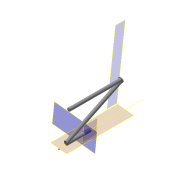
# Autodesk Inventor part: cellSTORM_lightpath
Saved by Autodesk Inventor 2022 (Build 260153000, 153)
## iProperties
Created: 2020-04-25
Part Number: cellSTORM_lightpath
Material: Generic
Document SubType Name: Modeling
Designer: diederichbenedict
Density: 1 g/cm^3
Appearance: Default
Author: diederichbenedict
Autodesk Inventor part; units mm, degrees
ref_plane "YZ Plane" through (0, 0, 0) normal (1, 0, 0) x (0, 1, 0)
ref_plane "XZ Plane" through (0, 0, 0) normal (0, 1, 0) x (-1, 0, 0)
ref_plane "XY Plane" through (0, 0, 0) normal (0, 0, 1) x (1, 0, 0)
ref_plane "Work Plane1" through (-18.0552, 1.9841, 10) normal (0, 0, -1) x (-0.994, 0.1092, 0)
ref_plane "Work Plane4" through (0, 0, 10) normal (-0.994, 0.1092, 0) x (-0.1092, -0.994, 0)
ref_plane "Work Plane3" through (-40.2485, 19.0101, 10) normal (-0.994, 0.1092, 0) x (-0.1092, -0.994, 0)
sketch "Sketch1" plane through (0, 0, 10) normal (-0.994, 0.1092, 0) x (-0.1092, -0.994, 0)
  line L0 (0, -10) -> (0, 30)
  line L1 (0, 30) -> (-50, -56.6025)
  line L2 (-50, -56.6025) -> (-50, 28.3975)
  line L3 (-7.1094, 32.5876) -> (7.1094, 27.4124)
  line L4 (-58.0583, -53.6696) -> (-41.9417, -59.5355)
  line L5 (-50, -56.6025) -> (-68.7133, -89.015)
  line L6 (-65.9988, -87.2149) -> (-113.9988, -87.2149)
  line L7 (-85.9997, -87.615) -> (-57.6047, -87.615)
  line L8 (-57.6047, -90.815) -> (-85.9997, -90.815)
  line L9 (-81.8462, -89.015) -> (-68.7133, -89.015)
  dimension "d0" = 40
  dimension "d1" = 100
  dimension "d2" = 30
  dimension "d3" = 85
  dimension "d4" = 30
  dimension "d6" = 70
  dimension "d19" = 1.4
  constraints: 21 end point, 2 midpoint, 2 parallel, 1 collinear, 1 horizontal, 1 vertical, 9 other
  measures "d0" distance of L0.end L0.start
  measures "d1" distance of L0.end L1.end
  measures "d2" angle of L1 L0
  measures "d3" distance of L1.end L2.end
  measures "d4" angle of L1 L2
  measures "d6" angle of L3 L0
  measures "d19" vertical distance of L5.end L7.end
ref_plane "Work Plane7" through (-18.0552, 1.9841, 10) normal (0, 0, -1) x (-0.994, 0.1092, 0)
sketch "Sketch3" plane through (-18.0552, 1.9841, 10) normal (0, 0, -1) x (-0.994, 0.1092, 0)
  circle A0 centre (-18.1638, 0) radius 11.5 projected
  circle A1 centre (-18.1638, 0) radius 2.5
  point P0 (-18.1638, 0)
  dimension "d7" = 5
  constraints: 1 centre point, 1 coincident
  measures "d7" diameter of A1
sweep "Sweep1" add profiles "Sketch3" path "Sketch1" path curves L0 L1 L2 contours A1
ref_plane "Work Plane8" through (-22.055, 95.458, -62.5) normal (-0.994, 0.1092, 0) x (-0.1092, -0.994, 0)
sketch "Sketch4" plane through (-22.055, 95.458, -62.5) normal (-0.994, 0.1092, 0) x (-0.1092, -0.994, 0)
  line L0 (44.9778, 100.8975) -> (39.9778, 100.8975) projected
  line L1 (42.4778, 15.8975) -> (42.4778, 15.8975) projected
  line L2 (42.4778, 15.8975) -> (42.4778, 15.8975) projected
  line L3 (42.4778, 15.8975) -> (42.4778, 15.8975) projected
  line L4 (42.4778, 15.8975) -> (42.4778, 15.8975) projected
  line L5 (92.4778, 102.5) -> (92.4778, 102.5) projected
  line L6 (92.4778, 102.5) -> (92.4778, 102.5) projected
  line L7 (92.4778, 102.5) -> (92.4778, 102.5) projected
  line L8 (92.4778, 102.5) -> (92.4778, 102.5) projected
  line L9 (94.9778, 62.5) -> (89.9778, 62.5) projected
  line L10 (56.4279, -3) -> (16.4279, -3) projected
  line L11 (39.9778, 6.5673) -> (39.9778, 100.8975) projected
  line L12 (44.9778, 25.2276) -> (44.9778, 100.8975) projected
  line L13 (94.9778, 111.8301) -> (44.9778, 25.2276) projected
  line L14 (89.9778, 93.1699) -> (39.9778, 6.5673) projected
  line L15 (89.9778, 62.5) -> (89.9778, 93.1699) projected
  line L16 (94.9778, 62.5) -> (94.9778, 111.8301) projected
  line L17 (34.8879, 19.8987) -> (57.029, 15.9946)
  line L18 (57.029, 15.9946) -> (43.097, -3.4007)
  line L19 (43.097, -3.4007) -> (27.2737, 11.5768)
  line L20 (27.2737, 11.5768) -> (33.0712, 21.6183)
  line L21 (34.8879, 19.8987) -> (33.0712, 21.6183)
  line L22 (80.9168, 101.8756) -> (102.3497, 98.0964)
  line L23 (102.3497, 98.0964) -> (104.1096, 108.0773)
  line L24 (104.1096, 108.0773) -> (90.6818, 110.445)
  line L25 (90.6818, 110.445) -> (80.9168, 101.8756)
  point P0 (92.4778, 62.5)
  dimension "d10" = 70
  dimension "d11" = 7
  dimension "d12" = 7
  constraints: 18 end point, 2 parallel, 1 perpendicular, 1 point on line
  measures "d10" angle of L17 L14
  measures "d11" distance from line of L17 L12.start
  measures "d12" distance from line of L22 L15.end
extrude "Extrusion1" cut sketch "Sketch4" against normal through all contours L17 L14 L11 | L11 L14 L17 L18 L10 L19 L20 L21 | L22 L25 L24 L13 | L13 L24 L16 L22 | L16 L24 L23 L22 | L18 L19 L10
sketch "Sketch5" plane through (5.4615, 49.7008, -43.9396) normal (0.019, 0.1726, -0.9848) x (-0.994, 0.1092, 0)
  ellipse E0 centre (0, -1.4169) end of major axis (0, -4.0774) minor radius 2.5 (-2.4054, -0.6919) -> (2.4054, -0.6919) ccw projected
  ellipse E1 centre (0, 0) end of major axis (0, 2.5386) minor radius 2.5 (2.4054, -0.6919) -> (-2.4054, -0.6919) ccw projected
  line L0 (-2.4054, -0.1127) -> (2.4054, -0.1127) projected
  circle A0 centre (0, -0.1127) radius 3.7871
  point P0 (0, -41.6104)
  constraints: 1 centre point, 4 other
extrude "Extrusion2" add sketch "Sketch5" against normal blind 1 contours E1 E0 A0 | E0 A0 E1
sketch "Sketch6" plane through (0.1524, 1.3871, 37.5831) normal (-0.019, -0.1726, 0.9848) x (0.994, -0.1092, 0)
  ellipse E0 centre (0, 0) end of major axis (0, -2.6604) minor radius 2.5 (2.4054, -0.7251) -> (-2.4054, -0.7251) ccw projected
  ellipse E1 centre (0, -1.4169) end of major axis (0, 1.1216) minor radius 2.5 (-2.4054, -0.7251) -> (2.4054, -0.7251) ccw projected
  line L0 (-2.4054, -0.1127) -> (2.4054, -0.1127) projected
  circle A0 centre (0, -0.1127) radius 3.2394
  point P0 (0, -7.9004)
  constraints: 1 centre point, 4 other
extrude "Extrusion3" add sketch "Sketch6" against normal blind 1 contours E1 A0 E0 | E0 E1 A0
ref_plane "Arbeitsebene10" through (0, 0, 0) normal (0.1092, 0.994, 0) x (0, 0, -1)
ref_plane "Arbeitsebene9" through (28.1562, 85.4859, 52.7288) normal (0.1092, 0.994, 0) x (0, 0, -1)
sketch "Skizze7" plane through (0, 0, 0) normal (1, 0, 0) x (0, 1, 0)
  ellipse E0 centre (1.916, 36.6615) end of major axis (-0.7027, 36.2019) minor radius 0.0475 (1.1885, 36.4876) -> (0.6825, 36.4876) ccw projected
  ellipse E1 centre (0, 40) end of major axis (2.487, 30.6701) minor radius 0.2639 (0.6825, 36.4876) -> (1.1885, 36.4876) ccw projected
  ellipse E2 centre (47.7849, -43.264) end of major axis (45.1662, -43.7236) minor radius 0.0475 (48.5123, -43.0901) -> (46.0809, -43.5264) ccw projected
  ellipse E3 centre (49.7008, -46.6025) end of major axis (52.1878, -55.9324) minor radius 0.2639 (49.0183, -43.0901) -> (48.5123, -43.0901) ccw projected
  ellipse E4 centre (47.7849, -43.264) end of major axis (45.1662, -43.7236) minor radius 0.0475 (46.5304, -43.5264) -> (49.0183, -43.0901) ccw projected
  ellipse E5 centre (48.3138, -44.1856) end of major axis (45.6952, -44.6452) minor radius 0.0475 (45.984, -44.5724) -> (46.2826, -44.5724) ccw projected
  line L0 (83.756, -77.615) -> (55.528, -77.615) projected
  line L1 (55.528, -80.815) -> (83.756, -80.815) projected
  line L2 (48.3138, -44.1856) -> (68.5318, -79.415)
  line L3 (68.5318, -79.415) -> (89.5946, -79.415)
  ellipse E6 centre (1.916, 36.6615) end of major axis (-0.7027, 36.2019) minor radius 0.0475 (1.1885, 36.4876) -> (0.6825, 36.4876) ccw projected
  ellipse E7 centre (0, 40) end of major axis (2.487, 30.6701) minor radius 0.2639 (0.6825, 36.4876) -> (1.1885, 36.4876) ccw projected
  ellipse E8 centre (47.7849, -43.264) end of major axis (45.1662, -43.7236) minor radius 0.0475 (48.5123, -43.0901) -> (46.0809, -43.5264) ccw projected
  ellipse E9 centre (49.7008, -46.6025) end of major axis (52.1878, -55.9324) minor radius 0.2639 (49.0183, -43.0901) -> (48.5123, -43.0901) ccw projected
  ellipse E10 centre (47.7849, -43.264) end of major axis (45.1662, -43.7236) minor radius 0.0475 (46.5304, -43.5264) -> (49.0183, -43.0901) ccw projected
  ellipse E11 centre (48.3138, -44.1856) end of major axis (45.6952, -44.6452) minor radius 0.0475 (45.984, -44.5724) -> (46.2826, -44.5724) ccw projected
  line L4 (4.5345, 37.1214) -> (47.2528, -37.3144) projected
  line L5 (2.448, 30.7118) -> (45.6953, -44.6455) projected
  point P0 (0, 0)
  dimension "d20" = 1.4
  constraints: 4 end point, 2 parallel, 16 other
  measures "d20" distance between parallel lines of L3 L1
ref_plane "Work Plane2" through (-1.6385, -14.9102, 10) normal (0, 0, 1) x (0.994, -0.1092, 0)
body "Solid1"
